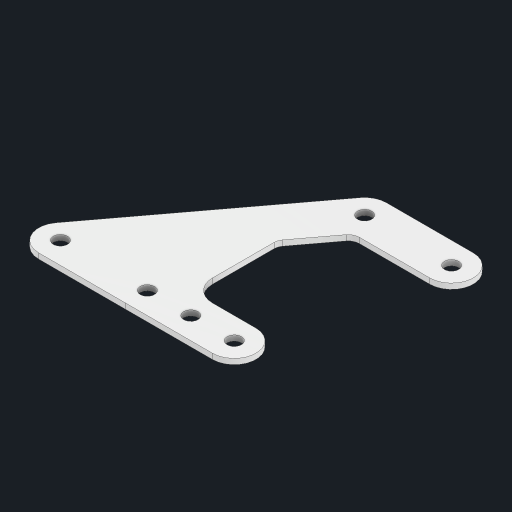
# Autodesk Inventor part: gusset
Saved by Autodesk Inventor 2024 (Build 280153000, 153)
## iProperties
Created: 2024-03-11
Part Number: gusset
Material: Acetal Resin, White
Document SubType Name: Modeling
Designer: Averey Ku
Density: 1.425 g/cm^3
Appearance: Smooth - White
Author: Averey Ku
Autodesk Inventor part; units mm, degrees
ref_plane "YZ Plane" through (0, 0, 0) normal (1, 0, 0) x (0, 1, 0)
ref_plane "XZ Plane" through (0, 0, 0) normal (0, 1, 0) x (-1, 0, 0)
ref_plane "XY Plane" through (0, 0, 0) normal (0, 0, 1) x (1, 0, 0)
sketch "main" plane through (0, 0, 0) normal (0, 0, 1) x (1, 0, 0)
  arc A0 (-6.1043, -28.9805) -> (-0.9888, -26.4406) centre (-6.0688, -22.6306) ccw
  arc A1 (-31.4687, -16.2806) -> (-31.4687, -28.9806) centre (-31.4688, -22.6306) ccw
  circle A2 centre (-6.0688, -22.6306) radius 2.0955
  circle A3 centre (-31.4688, -22.6306) radius 2.0955
  line L0 (-10.8313, -16.2806) -> (-31.4688, -16.2806)
  line L1 (-6.0331, -28.9805) -> (-31.4687, -28.9806)
  circle A4 centre (-6.0688, 28.169) radius 2.0955
  circle A5 centre (6.6312, 28.1694) radius 2.0955
  line L2 (0.2812, 15.4694) -> (0.2812, -2.5222)
  line L3 (37.1112, 24.3594) -> (-0.9888, -26.4406)
  line L4 (-18.7688, 21.8194) -> (-6.0688, 21.8194)
  arc A6 (0.2812, 15.4694) -> (-6.0688, 21.8194) centre (-6.0688, 15.4694) ccw
  arc A7 (-18.6975, 34.519) -> (-18.7688, 21.8194) centre (-18.7688, 28.1694) ccw
  line L5 (-18.6975, 34.519) -> (6.6312, 34.519)
  circle A8 centre (32.0312, 28.1694) radius 2.0955
  arc A9 (37.1112, 24.3594) -> (32.0311, 34.5194) centre (32.0312, 28.1694) ccw
  line L6 (6.6311, 34.519) -> (32.0311, 34.5194)
  circle A10 centre (-18.7688, 28.1694) radius 2.0956
  line L7 (-0.3538, -4.4272) -> (-8.2913, -15.0106)
  arc A11 (-10.8313, -16.2806) -> (-8.2913, -15.0106) centre (-10.8313, -13.1056) ccw
  arc A12 (-0.3538, -4.4272) -> (0.2812, -2.5222) centre (-2.8938, -2.5222) ccw
  point P0 (-4.0049, 2.2465)
  point P1 (0.2812, -3.5806)
  dimension "d0" = 4.191
  dimension "d1" = 4.191
  dimension "d2" = 12.7
  dimension "d4" = 6.35
  dimension "d7" = 6.35
  dimension "d8" = 25.4
  dimension "d9" = 3.175
  measures "d0" diameter of A4
  measures "d1" diameter of A8
  measures "d2" diameter of A0
  measures "d4" radius of A6
  measures "d7" radius of A9
  measures "d8" distance of A8.centre A5.centre
  measures "d9" radius of A11
sketch "Sketch1" plane through (0, 0, 0) normal (0, 1, 0) x (-1, 0, 0)
  arc A0 (-0.0356, -57.1495) -> (5.08, -54.6096) centre (0, -50.7996) ccw
  arc A1 (-25.4, -44.4496) -> (-25.4, -57.1496) centre (-25.4, -50.7996) ccw
  circle A2 centre (0, -50.7996) radius 2.0955
  circle A3 centre (-25.4, -50.7996) radius 2.0955
  line L0 (-4.7625, -44.4496) -> (-25.4, -44.4496)
  line L1 (0.0356, -57.1495) -> (-25.4, -57.1496)
  circle A4 centre (0, 0) radius 2.0955
  circle A5 centre (12.7, 0.0004) radius 2.0955
  line L2 (6.35, -12.6996) -> (6.35, -30.6913)
  line L3 (43.18, -3.8096) -> (5.08, -54.6096)
  line L4 (-12.7, -6.3496) -> (0, -6.3496)
  arc A6 (6.35, -12.6996) -> (0, -6.3496) centre (0, -12.6996) ccw
  arc A7 (-12.6287, 6.35) -> (-12.7, -6.3496) centre (-12.7, 0.0004) ccw
  line L5 (-12.6287, 6.35) -> (12.7, 6.35)
  circle A8 centre (38.1, 0.0004) radius 2.0955
  arc A9 (43.18, -3.8096) -> (38.0999, 6.3504) centre (38.1, 0.0004) ccw
  line L6 (12.6999, 6.35) -> (38.0999, 6.3504)
  circle A10 centre (-12.7, 0.0004) radius 2.0956
  line L7 (5.715, -32.5963) -> (-2.2225, -43.1796)
  arc A11 (-4.7625, -44.4496) -> (-2.2225, -43.1796) centre (-4.7625, -41.2746) ccw
  arc A12 (5.715, -32.5963) -> (6.35, -30.6913) centre (3.175, -30.6913) ccw
  point P0 (12.7, 6.35)
  point P1 (12.7, 6.35)
  constraints: 1 other
extrude "Extrusion1" add sketch "Sketch1" along normal blind 1.5875
body "Solid1"
